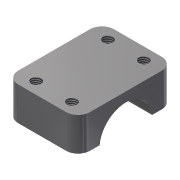
# Autodesk Inventor part: GARFO
Saved by Autodesk Inventor 2015 (Build 190159000, 159)
## iProperties
Created: 2016-08-09
Part Number: GARFO
Material: Aluminium AW-7020
Document SubType Name: Modeling
Designer: EriveltonDell
Density: 2.78 g/cm^3
Appearance: Stainless - Brushed
Mass: 1234.07 g
Surface Area: 731.335 cm^2
Volume: 443.911 cm^3
Author: EriveltonDell
Autodesk Inventor part; units mm, degrees
ref_plane "YZ Plane" through (0, 0, 0) normal (1, 0, 0) x (0, 1, 0)
ref_plane "XZ Plane" through (0, 0, 0) normal (0, 1, 0) x (-1, 0, 0)
ref_plane "XY Plane" through (0, 0, 0) normal (0, 0, 1) x (1, 0, 0)
sketch "Sketch4" plane through (0, 0, 0) normal (0, 0, 1) x (1, 0, 0)
  line L0 (0, 0) -> (-30, 0)
  line L1 (-30, 0) -> (-30, 40)
  line L2 (-30, 40) -> (0, 40)
  line L3 (0, 40) -> (0, 0)
  dimension "d37" = 30
  dimension "d38" = 40
  constraints: 8 end point, 2 parallel, 1 horizontal, 1 perpendicular
  measures "d37" distance of L1.end L2.end
  measures "d38" distance of L0.end L1.end
extrude "Extrusion2" add sketch "Sketch4" along normal blind 14
hole "Hole3" at (-22.5, 35, 14) direction (0, 0, -1) diameter 4.134 depth 14.2 tip angle 118 thread size "M5x0.8" class "6H" standard "ISO Metric profile"
hole "Hole4" at (-7.5, 35, 14) direction (0, 0, -1) diameter 4.134 depth 14.2 tip angle 118 thread size "M5x0.8" class "6H" standard "ANSI Metric M Profile"
hole "Hole5" at (-7.5, 5, 14) direction (0, 0, -1) diameter 4.134 depth 14.2 tip angle 118 thread size "M5x0.8" class "6H" standard "ANSI Metric M Profile"
hole "Hole6" at (-22.5, 5, 14) direction (0, 0, -1) diameter 4.134 depth 14.2 tip angle 118 thread size "M5x0.8" class "6H" standard "ANSI Metric M Profile"
hole "Hole7" at (0, 20, -1) direction (-1, 0, 0) diameter 22 end through all
fillet "Fillet1" radius 5 4 edges at (-30, 40, 7) (0, 40, 7) (0, 0, 7) (-30, 0, 7)
body "Solid2"
